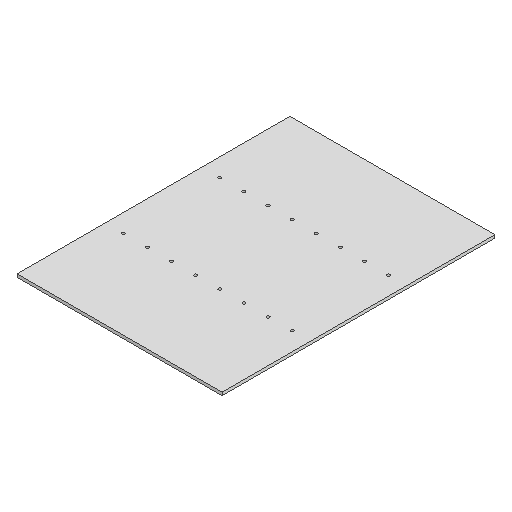
# Autodesk Inventor part: MotorAttachementPlate
Saved by Autodesk Inventor 2024 (Build 280153000, 153)
## iProperties
Created: 2024-02-14
Part Number: MotorAttachementPlate
Material: Generic
Document SubType Name: Modeling
Designer: seene
Density: 1 g/cm^3
Appearance: Default
Author: seene
Autodesk Inventor part; units mm, degrees
ref_plane "YZ Plane" through (0, 0, 0) normal (1, 0, 0) x (0, 1, 0)
ref_plane "XZ Plane" through (0, 0, 0) normal (0, 1, 0) x (-1, 0, 0)
ref_plane "XY Plane" through (0, 0, 0) normal (0, 0, 1) x (1, 0, 0)
sketch "Sketch1" plane through (0, 0, 0) normal (0, 1, 0) x (-1, 0, 0)
  line L0 (-215.9, 287.3375) -> (215.9, 287.3375)
  line L1 (215.9, 287.3375) -> (215.9, -287.3375)
  line L2 (215.9, -287.3375) -> (-215.9, -287.3375)
  line L3 (-215.9, -287.3375) -> (-215.9, 287.3375)
  line L4 (-215.9, 287.3375) -> (215.9, -287.3375) construction
  line L5 (215.9, 287.3375) -> (-215.9, -287.3375) construction
  line L6 (330.2, 88.9) -> (-330.2, 88.9) construction
  line L7 (-330.2, 88.9) -> (-330.2, 114.3) construction
  line L8 (-330.2, 114.3) -> (330.2, 114.3) construction
  line L9 (330.2, 114.3) -> (330.2, 88.9) construction
  circle A0 centre (228.6, 101.6) radius 3.175
  line L10 (330.2, 101.6) -> (228.6, 101.6) construction
  line L11 (215.9, 0) -> (-215.9, 0) construction
  circle A1 centre (177.8, 101.6) radius 3.175
  circle A2 centre (127, 101.6) radius 3.175
  circle A3 centre (76.2, 101.6) radius 3.175
  circle A4 centre (25.4, 101.6) radius 3.175
  circle A5 centre (-25.4, 101.6) radius 3.175
  circle A6 centre (-76.2, 101.6) radius 3.175
  circle A7 centre (-127, 101.6) radius 3.175
  circle A8 centre (-177.8, 101.6) radius 3.175
  circle A9 centre (-228.6, 101.6) radius 3.175
  line L12 (330.2, -88.9) -> (-330.2, -88.9) construction
  line L13 (-330.2, -88.9) -> (-330.2, -114.3) construction
  line L14 (-330.2, -114.3) -> (330.2, -114.3) construction
  line L15 (330.2, -114.3) -> (330.2, -88.9) construction
  circle A10 centre (228.6, -101.6) radius 3.175
  circle A11 centre (177.8, -101.6) radius 3.175
  circle A12 centre (127, -101.6) radius 3.175
  circle A13 centre (76.2, -101.6) radius 3.175
  circle A14 centre (25.4, -101.6) radius 3.175
  circle A15 centre (-25.4, -101.6) radius 3.175
  circle A16 centre (-76.2, -101.6) radius 3.175
  circle A17 centre (-127, -101.6) radius 3.175
  circle A18 centre (-177.8, -101.6) radius 3.175
  circle A19 centre (-228.6, -101.6) radius 3.175
  point P0 (0, 0)
  point P1 (-330.2, 101.6)
  dimension "d0" = 431.8
  dimension "d4" = 25.4
  dimension "d7" = 114.3
  dimension "d8" = 6.35
  dimension "d9" = 101.6
  dimension "d10" = 660.4
  dimension "d11" = 330.2
  dimension "d16" = 50.8
  dimension "d22" = 173.0375
  constraints: 32 end point, 20 centre point, 14 symmetric about line, 6 midpoint, 4 horizontal, 4 parallel, 2 perpendicular, 28 other
  measures "d0" distance of L1.end L2.end
  measures "d4" distance of L6.end L7.end
  measures "d7" distance from line of point (0, 0) L8
  measures "d8" diameter of A0
  measures "d9" distance of L10.end L10.start
  measures "d10" distance from line of point (-330.2, 101.6) L9
  measures "d11" distance from line of L9 point (0, 0)
  measures "d16" distance of L10.end A1.centre
  measures "d22" distance between parallel lines of L0 L8
extrude "Extrusion1" add sketch "Sketch1" along normal blind 6.35 contours L0 L1 L2 L3
equation "\"d7\" = 0.5 * d6"
equation "\"d11\" = 0.5 * d10"
equation "\"d6\" = 228.6"
body "Solid1"
